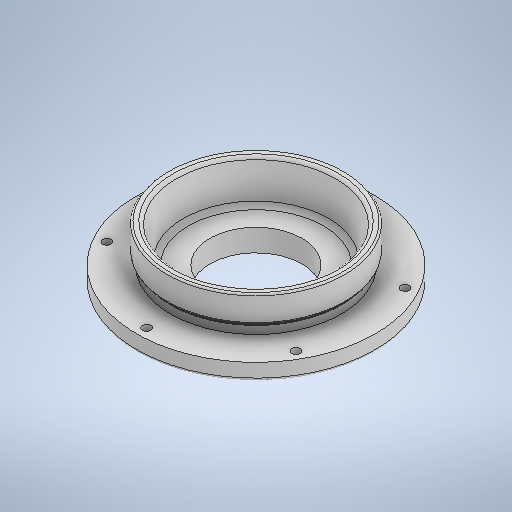
# Autodesk Inventor part: 40_Nap_o_thung
Saved by Autodesk Inventor 2025.2 (Build 292293000, 293)
## iProperties
Created: 2024-11-27
Part Number: 40_Nap_o_thung
Material: Generic
Document SubType Name: Modeling
Designer: hongquan
Density: 1 g/cm^3
Appearance: Default
Author: hongquan
Autodesk Inventor part; units mm, degrees
ref_plane "YZ Plane" through (0, 0, 0) normal (1, 0, 0) x (0, 1, 0)
ref_plane "XZ Plane" through (0, 0, 0) normal (0, 1, 0) x (-1, 0, 0)
ref_plane "XY Plane" through (0, 0, 0) normal (0, 0, 1) x (1, 0, 0)
sketch "Sketch1" plane through (0, 0, 0) normal (1, 0, 0) x (0, 1, 0)
  line L0 (0, 0) -> (0, -13)
  line L1 (0, -13) -> (0, -13)
  line L2 (3, -16.8284) -> (3, -41)
  line L3 (5, -43) -> (13, -43)
  line L4 (13, -43) -> (13, -23)
  line L5 (13, -23) -> (17.5858, -23)
  line L6 (18.2929, -23.2929) -> (19.7071, -24.7071)
  line L7 (20.4142, -25) -> (34, -25)
  line L8 (35, -24) -> (35, -21.5965)
  line L9 (13, -12.6053) -> (13, 0)
  arc A0 (34, -25) -> (35, -24) centre (34, -24) ccw
  arc A1 (19.7071, -24.7071) -> (20.4142, -25) centre (20.4142, -24) ccw
  arc A2 (18.2929, -23.2929) -> (17.5858, -23) centre (17.5858, -24) ccw
  arc A3 (3, -41) -> (5, -43) centre (5, -41) ccw
  line L10 (0, -13) -> (2.4142, -15.4142)
  arc A4 (3, -16.8284) -> (2.4142, -15.4142) centre (1, -16.8284) ccw
  line L11 (33.4432, -19.6462) -> (15.3351, -15.5307)
  line L12 (13, 0) -> (0, 0)
  arc A5 (35, -21.5965) -> (33.4432, -19.6462) centre (33, -21.5965) ccw
  arc A6 (13, -12.6053) -> (15.3351, -15.5307) centre (16, -12.6053) ccw
  line L13 (64.2413, 27) -> (-63.4715, 27)
  point P0 (3, -13)
  point P1 (3, -43)
  point P2 (18, -23)
  point P3 (20, -25)
  point P4 (35, -25)
  point P5 (35, -18)
  point P6 (13, -18)
  dimension "d0" = 32
  dimension "d1" = 10
  dimension "d2" = 13
  dimension "d3" = 3
  dimension "d5" = 20
  dimension "d6" = 5
  dimension "d7" = 2
  dimension "d8" = 2
  dimension "d9" = 22
  dimension "d10" = 7
  dimension "d14" = 1
  dimension "d15" = 1
  dimension "d16" = 2
  dimension "d17" = 2
  dimension "d18" = 2
  dimension "d19" = 3
  dimension "d20" = 140
  constraints: 28 end point, 14 point on circle, 14 tangent, 12 point on line, 7 centre point, 6 perpendicular, 3 horizontal, 1 equal radius, 1 parallel, 1 vertical, 4 other
  measures "d0" distance between parallel lines of L2 L8
  measures "d1" distance of point (3, -43) L3.end
  measures "d2" distance of L0.start L0.end
  measures "d3" distance of L0.end point (3, -13)
  measures "d5" distance of L3.end L4.end
  measures "d6" distance of L4.end point (18, -23)
  measures "d7" distance between parallel lines of L7 L5
  measures "d8" horizontal distance of point (18, -23) point (20, -25)
  measures "d9" distance of point (35, -18) point (13, -18)
  measures "d10" distance of point (35, -25) point (35, -18)
  measures "d14" radius of A0
  measures "d15" radius of A1
  measures "d16" radius of A3
  measures "d17" radius of A4
  measures "d18" radius of A5
  measures "d19" radius of A6
  measures "d20" diameter of L3 L13
revolve "Revolution1" add sketch "Sketch1" angle 360 about axis through (0, 64.2413, 27) along (0, -1, 0)
sketch "Sketch2" plane through (0, 3, 27) normal (0, -1, 0) x (1, 0, 0)
  circle A0 centre (0, 0) radius 64 construction
  point P0 (0, -27)
  point P1 (0, 64)
  point P2 (0, 64)
  dimension "d22" = 128
  constraints: 1 coincident, 1 vertical alignment, 2 other
hole "Hole1" at (0, 3, 91) direction (0, 1, 0) diameter 5 end through all
chamfer "Chamfer1" distance 0.5 angle 45 1 edges at (0, 3, 93.5)
pattern_circular "Circular Pattern1" count 6 over 360 about axis through (0, 9, 27) along (0, -1, 0) of "Hole1"
body "Solid1"
